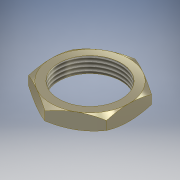
# Autodesk Inventor part: Nut_M8x0.5_2mm
Saved by Autodesk Inventor 2018 (Build 220112000, 112)
## iProperties
Created: 2018-06-04
Part Number: Nut_M8x0.5_2mm
Material: Brass, Soft Yellow
Document SubType Name: Modeling
Designer: Bradley
Density: 8.47 g/cm^3
Appearance: Nickel
Author: Bradley
Autodesk Inventor part; units mm, degrees
ref_plane "YZ Plane" through (0, 0, 0) normal (1, 0, 0) x (0, 1, 0)
ref_plane "XZ Plane" through (0, 0, 0) normal (0, 1, 0) x (-1, 0, 0)
ref_plane "XY Plane" through (0, 0, 0) normal (0, 0, 1) x (1, 0, 0)
sketch "Sketch1" plane through (0, 0, 0) normal (0, 1, 0) x (-1, 0, 0)
  line L0 (0, 1) -> (0, -1)
  line L1 (-4, 1) -> (-4, -1)
  line L2 (-4, -1) -> (-5, -1)
  line L3 (-5, -1) -> (-6.7321, 0)
  line L4 (-6.7321, 0) -> (-5, 1)
  line L5 (-5, 1) -> (-4, 1)
  point P0 (0, 0)
  point P1 (0, 0)
  dimension "d0" = 10
  dimension "d1" = 8
  dimension "d2" = 2
  dimension "d4" = 30
  constraints: 12 end point, 2 equal length, 2 point on line, 2 vertical, 1 coincident, 1 midpoint, 1 parallel, 1 perpendicular
  measures "d0" diameter of L4.end L0
  measures "d1" diameter of L1 L0
  measures "d2" distance of L0.start L0.end
  measures "d4" angle of L2 L3
revolve "Revolution1" add sketch "Sketch1" angle 360 about axis through (0, 0, 1) along (0, 0, -1)
sketch "Sketch2" plane through (0, 0, 1) normal (0, 0, 1) x (1, 0, 0)
  circle A0 centre (0, 0) radius 4 projected
  circle A1 centre (0, 0) radius 5 projected
  line L0 (0, 5.7735) -> (5, 2.8868)
  line L1 (5, 2.8868) -> (5, -2.8868)
  line L2 (5, -2.8868) -> (0, -5.7735)
  line L3 (0, -5.7735) -> (-5, -2.8868)
  line L4 (-5, -2.8868) -> (-5, 2.8868)
  line L5 (-5, 2.8868) -> (0, 5.7735)
  point P0 (0, 0)
  constraints: 12 end point, 1 coincident, 1 tangent, 1 vertical, 13 other
extrude "Extrusion1" cut sketch "Sketch2" against normal through all keep common part
thread "Thread1" size "M8x0.5" class "6H" standard "ANSI Metric M Profile" full length
body "Solid1"
